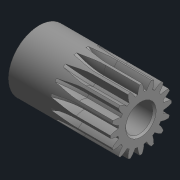
# Autodesk Inventor part: SS1-16_On
Saved by Autodesk Inventor 2022 (Build 260153000, 153)
## iProperties
Part Number: SS1-16_On
Material: 一般
Catalog Web Link: www.cadenas.de
Description: Steel, Spur Gears (SS)-
Vendor: KHK
Document SubType Name: Modeling
Designer: partserver
Manufacturer: KHK
Mass: 5.26127 g
Surface Area: 34.7656 cm^2
Volume: 5.26127 cm^3
Density: 1 g/cm^3
Appearance: PSOLRGB-175-175-175
Category: PARTsolutions
Company: KHK
PSOL_IDENT_0: {$CADENAS_DATA\23d-libs\khk\spur_gears\steel_spur_gears_ss.prj},181 {VTYP=3D},{NB=SS1-16_On},{LINA=S
PSOL_IDENT_1: S1-16},{NN=Steel, Spur Gears (SS)},{DATE=04.11.2021 04:47:04},{GEOMDATE=02.07.2021 05:38:00},{VERSIO
PSOL_IDENT_2: N=},{LINEID=5340},{WBVAR=TOOTH,HT},{WBNUMERIC=}  {NB=SS1-16_On},{LINA=SS1-16},{KT=DUMMY},{CN=SS1-16}
PSOL_IDENT_3: ,{CN1=SS1-16},{ST=},{M=1},{MX=1.000},{Z=16},{A=8},{B=18.0},{C=16.0},{D=18.0},{E=10},{F=20},{G=30},{H=
PSOL_IDENT_4: 0},{I=0},{K=0},{L=0.0},{M1=0},{J=0.0},{S=S3},{R=1},{N=0.5},{L1=0.5},{L2=0.5},{M11=0},{X=0},{XX=0},{K
PSOL_IDENT_5: EY=1},{CBD1=0.0},{CBD2=0.0},{TOOTH=On},{HTX='','without','H','with'},{HT=},{NEW=0}
NB: SS1-16_On
NN: Steel, Spur Gears (SS)
NBSYN: $CN._$TOOTH.
LINA: SS1-16
CATALOG: KHK
CN: SS1-16
M: 1
Z: 16
A: 8
B: 18
C: 16
D: 18
E: 10
F: 20
G: 30
H: 0
I: 0
K: 0
L: 0
M1: 0
J: 0
S: S3
TOOTH: On
HT: without
NEW: 0
SUPPLIER: KHK
ARTICLENO: SS1-16_On
BOMINFO: SS1-16
CREATOR: CADENAS GmbH
Title: SS1-16
Author: Cadenas PARTsolutions
Autodesk Inventor part; units mm, degrees
ref_plane "YZ Plane" through (0, 0, 0) normal (1, 0, 0) x (0, 1, 0)
ref_plane "XZ Plane" through (0, 0, 0) normal (0, 1, 0) x (-1, 0, 0)
ref_plane "XY Plane" through (0, 0, 0) normal (0, 0, 1) x (1, 0, 0)
sketch "Sketch_1" plane through (0, 0, 0) normal (0, 0, 1) x (1, 0, 0)
  line L0 (30, 0) -> (0, 0)
  line L1 (0, 4.5) -> (0.5, 4)
  line L2 (0.5, 4) -> (29.5, 4)
  line L3 (29.5, 4) -> (30, 4.5)
  line L4 (30, 4.5) -> (30, 9)
  line L5 (30, 9) -> (0, 9)
  line L6 (0, 9) -> (0, 4.5)
  constraints: 14 end point
revolve "Revolution1" add sketch "Sketch_1" angle 360 about axis through (30, 0, 0) along (1, 0, 0)
sketch "Sketch_4" plane through (0, 0, 0) normal (1, 0, 0) x (0, 1, 0)
  line L0 (18, 18) -> (-18, 18)
  line L1 (-18, 18) -> (-18, -18)
  line L2 (-18, -18) -> (18, -18)
  line L3 (18, -18) -> (18, 18)
  arc A0 (0.3533, 8.9931) -> (-0.3533, 8.9931) centre (0, 0) ccw
  arc A1 (-0.3533, 8.9931) -> (-0.9248, 6.6863) centre (5.0695, 6.4254) ccw
  arc A2 (-0.9248, 6.6863) -> (-1.7043, 6.5313) centre (0, 0) ccw
  arc A3 (-1.7043, 6.5313) -> (-3.1151, 8.4437) centre (-7.1425, 3.9963) ccw
  arc A4 (-3.1151, 8.4437) -> (-3.7679, 8.1733) centre (0, 0) ccw
  arc A5 (-3.7679, 8.1733) -> (-3.4132, 5.8235) centre (2.2247, 7.8763) ccw
  arc A6 (-3.4132, 5.8235) -> (-4.074, 5.3819) centre (0, 0) ccw
  arc A7 (-4.074, 5.3819) -> (-6.1092, 6.6089) centre (-8.1281, 0.9588) ccw
  arc A8 (-6.1092, 6.6089) -> (-6.6089, 6.1092) centre (0, 0) ccw
  arc A9 (-6.6089, 6.1092) -> (-5.3819, 4.074) centre (-0.9588, 8.1281) ccw
  arc A10 (-5.3819, 4.074) -> (-5.8235, 3.4132) centre (0, 0) ccw
  arc A11 (-5.8235, 3.4132) -> (-8.1733, 3.7679) centre (-7.8763, -2.2247) ccw
  arc A12 (-8.1733, 3.7679) -> (-8.4437, 3.1151) centre (0, 0) ccw
  arc A13 (-8.4437, 3.1151) -> (-6.5313, 1.7043) centre (-3.9963, 7.1425) ccw
  arc A14 (-6.5313, 1.7043) -> (-6.6863, 0.9248) centre (0, 0) ccw
  arc A15 (-6.6863, 0.9248) -> (-8.9931, 0.3533) centre (-6.4254, -5.0695) ccw
  arc A16 (-8.9931, 0.3533) -> (-8.9931, -0.3533) centre (0, 0) ccw
  arc A17 (-8.9931, -0.3533) -> (-6.6863, -0.9248) centre (-6.4254, 5.0695) ccw
  arc A18 (-6.6863, -0.9248) -> (-6.5313, -1.7043) centre (0, 0) ccw
  arc A19 (-6.5313, -1.7043) -> (-8.4437, -3.1151) centre (-3.9963, -7.1425) ccw
  arc A20 (-8.4437, -3.1151) -> (-8.1733, -3.7679) centre (0, 0) ccw
  arc A21 (-8.1733, -3.7679) -> (-5.8235, -3.4132) centre (-7.8763, 2.2247) ccw
  arc A22 (-5.8235, -3.4132) -> (-5.3819, -4.074) centre (0, 0) ccw
  arc A23 (-5.3819, -4.074) -> (-6.6089, -6.1092) centre (-0.9588, -8.1281) ccw
  arc A24 (-6.6089, -6.1092) -> (-6.1092, -6.6089) centre (0, 0) ccw
  arc A25 (-6.1092, -6.6089) -> (-4.074, -5.3819) centre (-8.1281, -0.9588) ccw
  arc A26 (-4.074, -5.3819) -> (-3.4132, -5.8235) centre (0, 0) ccw
  arc A27 (-3.4132, -5.8235) -> (-3.7679, -8.1733) centre (2.2247, -7.8763) ccw
  arc A28 (-3.7679, -8.1733) -> (-3.1151, -8.4437) centre (0, 0) ccw
  arc A29 (-3.1151, -8.4437) -> (-1.7043, -6.5313) centre (-7.1425, -3.9963) ccw
  arc A30 (-1.7043, -6.5313) -> (-0.9248, -6.6863) centre (0, 0) ccw
  arc A31 (-0.9248, -6.6863) -> (-0.3533, -8.9931) centre (5.0695, -6.4254) ccw
  arc A32 (-0.3533, -8.9931) -> (0.3533, -8.9931) centre (0, 0) ccw
  arc A33 (0.3533, -8.9931) -> (0.9248, -6.6863) centre (-5.0695, -6.4254) ccw
  arc A34 (0.9248, -6.6863) -> (1.7043, -6.5313) centre (0, 0) ccw
  arc A35 (1.7043, -6.5313) -> (3.1151, -8.4437) centre (7.1425, -3.9963) ccw
  arc A36 (3.1151, -8.4437) -> (3.7679, -8.1733) centre (0, 0) ccw
  arc A37 (3.7679, -8.1733) -> (3.4132, -5.8235) centre (-2.2247, -7.8763) ccw
  arc A38 (3.4132, -5.8235) -> (4.074, -5.3819) centre (0, 0) ccw
  arc A39 (4.074, -5.3819) -> (6.1092, -6.6089) centre (8.1281, -0.9588) ccw
  arc A40 (6.1092, -6.6089) -> (6.6089, -6.1092) centre (0, 0) ccw
  arc A41 (6.6089, -6.1092) -> (5.3819, -4.074) centre (0.9588, -8.1281) ccw
  arc A42 (5.3819, -4.074) -> (5.8235, -3.4132) centre (0, 0) ccw
  arc A43 (5.8235, -3.4132) -> (8.1733, -3.7679) centre (7.8763, 2.2247) ccw
  arc A44 (8.1733, -3.7679) -> (8.4437, -3.1151) centre (0, 0) ccw
  arc A45 (8.4437, -3.1151) -> (6.5313, -1.7043) centre (3.9963, -7.1425) ccw
  arc A46 (6.5313, -1.7043) -> (6.6863, -0.9248) centre (0, 0) ccw
  arc A47 (6.6863, -0.9248) -> (8.9931, -0.3533) centre (6.4254, 5.0695) ccw
  arc A48 (8.9931, -0.3533) -> (8.9931, 0.3533) centre (0, 0) ccw
  arc A49 (8.9931, 0.3533) -> (6.6863, 0.9248) centre (6.4254, -5.0695) ccw
  arc A50 (6.6863, 0.9248) -> (6.5313, 1.7043) centre (0, 0) ccw
  arc A51 (6.5313, 1.7043) -> (8.4437, 3.1151) centre (3.9963, 7.1425) ccw
  arc A52 (8.4437, 3.1151) -> (8.1733, 3.7679) centre (0, 0) ccw
  arc A53 (8.1733, 3.7679) -> (5.8235, 3.4132) centre (7.8763, -2.2247) ccw
  arc A54 (5.8235, 3.4132) -> (5.3819, 4.074) centre (0, 0) ccw
  arc A55 (5.3819, 4.074) -> (6.6089, 6.1092) centre (0.9588, 8.1281) ccw
  arc A56 (6.6089, 6.1092) -> (6.1092, 6.6089) centre (0, 0) ccw
  arc A57 (6.1092, 6.6089) -> (4.074, 5.3819) centre (8.1281, 0.9588) ccw
  arc A58 (4.074, 5.3819) -> (3.4132, 5.8235) centre (0, 0) ccw
  arc A59 (3.4132, 5.8235) -> (3.7679, 8.1733) centre (-2.2247, 7.8763) ccw
  arc A60 (3.7679, 8.1733) -> (3.1151, 8.4437) centre (0, 0) ccw
  arc A61 (3.1151, 8.4437) -> (1.7043, 6.5313) centre (7.1425, 3.9963) ccw
  arc A62 (1.7043, 6.5313) -> (0.9248, 6.6863) centre (0, 0) ccw
  arc A63 (0.9248, 6.6863) -> (0.3533, 8.9931) centre (-5.0695, 6.4254) ccw
  constraints: 128 point on circle, 64 centre point, 8 end point
extrude "Extrusion1" cut sketch "Sketch_4" along normal blind 10
sketch "Sketch_6" plane through (10, 0, 0) normal (1, 0, 0) x (0, 0, -1)
  line L0 (-24.3406, 16.2639) -> (-4.0384, 20.3023)
  arc A0 (-1.7043, 6.5313) -> (-3.2688, 8.5783) centre (-7.1425, 3.9963) ccw
  arc A1 (-0.9248, 6.6863) -> (-1.7043, 6.5313) centre (0, 0) ccw
  arc A2 (-0.2628, 9.1762) -> (-0.9248, 6.6863) centre (5.0695, 6.4254) ccw
  arc A3 (-0.2628, 9.1762) -> (-3.2688, 8.5783) centre (0, 0) ccw
  constraints: 8 point on circle, 4 centre point, 2 end point
revolve "Revolution2" cut sketch "Sketch_6" angle 40 about axis through (10, 16.2639, 24.3406) along (0, -0.1950903, 0.9807853)
pattern_circular "Circular Pattern1" count 16 over 360 about axis through (10, 0, 0) along (1, 0, 0) of "Revolution2"
body "Solid1"
